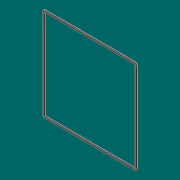
# Autodesk Inventor part: frontBackORing
Saved by Autodesk Inventor 2016 (Build 200138000, 138)
## iProperties
Created: 2015-10-19
Part Number: frontBackORing
Material: Rubber
Document SubType Name: Modeling
Designer: Sawaiz
Density: 0.93 g/cm^3
Appearance: Rubber - Black
Author: Sawaiz
Autodesk Inventor part; units mm, degrees
ref_plane "YZ Plane" through (0, 0, 0) normal (1, 0, 0) x (0, 1, 0)
ref_plane "XZ Plane" through (0, 0, 0) normal (0, 1, 0) x (-1, 0, 0)
ref_plane "XY Plane" through (0, 0, 0) normal (0, 0, 1) x (1, 0, 0)
sketch "Sketch1" plane through (0, 0, 0) normal (1, 0, 0) x (0, 1, 0)
  line L0 (-52.3875, -52.3875) -> (52.3875, -52.3875)
  line L1 (52.3875, -52.3875) -> (52.3875, 52.3875)
  line L2 (52.3875, 52.3875) -> (-52.3875, 52.3875)
  line L3 (-52.3875, 52.3875) -> (-52.3875, -52.3875)
  line L4 (-52.3875, -52.3875) -> (52.3875, 52.3875) construction
  line L5 (52.3875, -52.3875) -> (-52.3875, 52.3875) construction
  line L6 (-55.5625, 55.5625) -> (55.5625, 55.5625)
  line L7 (55.5625, 55.5625) -> (55.5625, -55.5625)
  line L8 (55.5625, -55.5625) -> (-55.5625, -55.5625)
  line L9 (-55.5625, -55.5625) -> (-55.5625, 55.5625)
  point P0 (0, 0)
  dimension "d0" = 104.775
  dimension "d1" = 104.775
  dimension "d2" = 3.175
  constraints: 20 end point, 4 parallel, 2 midpoint, 2 perpendicular, 1 horizontal, 3 other
  measures "d0" distance of L2.end L1.end
  measures "d1" distance of L0.end L1.end
  measures "d2" distance between parallel lines of L2 L6
extrude "Extrusion1" add sketch "Sketch1" along normal blind 1.905
fillet "Fillet1" radius 0.7937 16 edges at (1.905, 0, 55.5625) (0, 0, 55.5625) (1.905, 0, 52.3875) (0, 0, 52.3875) (1.905, 52.3875, 0) (1.905, 55.5625, 0) (0, 52.3875, 0) (0, 55.5625, 0) (1.905, 0, -55.5625) (1.905, 0, -52.3875) (0, 0, -55.5625) (0, 0, -52.3875) (0, -52.3875, 0) (1.905, -52.3875, 0) (0, -55.5625, 0) (1.905, -55.5625, 0)
fillet "Fillet2" radius 3.175 12 edges at (0.9525, 55.5625, 55.5625) (0.2325, 55.33, 55.33) (1.6725, 55.33, 55.33) (0.9525, -55.5625, 55.5625) (0.2325, -55.33, 55.33) (1.6725, -55.33, 55.33) (1.6725, -55.33, -55.33) (0.2325, -55.33, -55.33) (0.9525, -55.5625, -55.5625) (0.9525, 55.5625, -55.5625) (0.2325, 55.33, -55.33) (1.6725, 55.33, -55.33)
equation "\"d0\" = 0.25 * frontBackORingID"
equation "\"d1\" = 0.25 * frontBackORingID"
equation "\"d2\" = oRingWidth"
equation "\"d5\" = 0.25 * oRingWidth"
equation "\"d6\" = oRingWidth"
equation "\"acrylicThickness\" = 6.35"
equation "\"height\" = 101.6"
equation "\"width\" = 101.6"
equation "\"depth\" = 101.6"
equation "\"mirrorAngle\" = 5deg"
equation "\"detectorWidth\" = 52"
equation "\"detectorHeight\" = 52"
equation "\"mirrorThickness\" = 3"
equation "\"fresnelThickness\" = 0.1"
equation "\"focalLength\" = 76.2"
equation "\"ior\" = 1.49"
equation "\"centerThickness\" = 1.524"
equation "\"fresnelAngle\" = 90deg"
equation "\"fresnelEffectiveDiameter\" = 76.2"
equation "\"mirrorSuppourtWidth\" = 38.1"
equation "\"backGrooveBit\" = 4.8006"
equation "\"sensorHolderWidth\" = 88.9"
equation "\"sensorHolderHeight\" = 88.9"
equation "\"sensorHolderSensorHeight\" = 53.975"
equation "\"sensorHolderSensorWidth\" = 53.975"
equation "\"oRingWidth\" = 3.175"
equation "\"sensorHolderORingID\" = 203.2"
equation "\"sensorHolderFlushORingID\" = 254"
equation "\"frontBackORingID\" = 419.1"
equation "\"topBottomHorizontalMirrorGroove\" = 12.7"
equation "\"backMirrorGroove\" = 6.35"
equation "\"mirrorGroove\" = 19.05"
equation "\"fresnelChamfer\" = 6.35"
equation "\"mirrorGrooveFillet\" = 6.35"
equation "\"mirrorGrooveDrill\" = 6.35"
equation "\"mirrorGrooveMill\" = 3.175"
body "Solid1"
